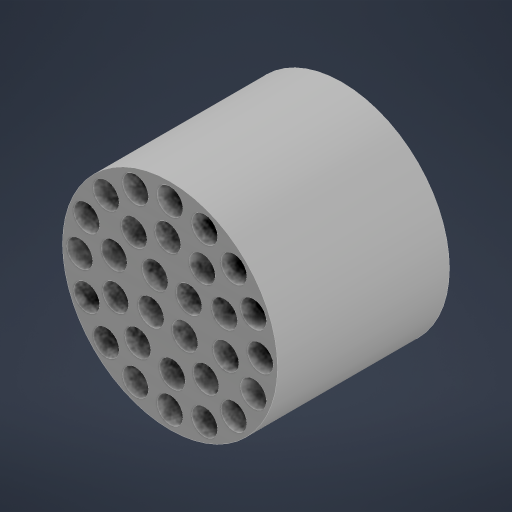
# Autodesk Inventor part: Membaranacentral
Saved by Autodesk Inventor 2024 (Build 280153000, 153)
## iProperties
Created: 2020-11-27
Part Number: Membaranacentral
Material: Plástico PET
Document SubType Name: Modeling
Designer: Tania Rios
Density: 1.541 g/cm^3
Appearance: Gris claro
Mass: 167.995 g
Surface Area: 1418.19 cm^2
Volume: 109.017 cm^3
Author: Tania Rios
Autodesk Inventor part; units mm, degrees
ref_plane "YZ Plane" through (0, 0, 0) normal (1, 0, 0) x (0, 1, 0)
ref_plane "XZ Plane" through (0, 0, 0) normal (0, 1, 0) x (-1, 0, 0)
ref_plane "XY Plane" through (0, 0, 0) normal (0, 0, 1) x (1, 0, 0)
sketch "Boceto1" plane through (0, 0, 0) normal (0, 0, 1) x (1, 0, 0)
  circle A0 centre (0, 0) radius 12.5
  circle A1 centre (0, 10.5) radius 1.5
  circle A2 centre (-4.0182, 9.7007) radius 1.5
  circle A3 centre (-7.4246, 7.4246) radius 1.5
  circle A4 centre (-9.7007, 4.0182) radius 1.5
  circle A5 centre (-10.5, 0) radius 1.5
  circle A6 centre (-9.7007, -4.0182) radius 1.5
  circle A7 centre (-7.4246, -7.4246) radius 1.5
  circle A8 centre (-4.0182, -9.7007) radius 1.5
  circle A9 centre (0, -10.5) radius 1.5
  circle A10 centre (4.0182, -9.7007) radius 1.5
  circle A11 centre (7.4246, -7.4246) radius 1.5
  circle A12 centre (9.7007, -4.0182) radius 1.5
  circle A13 centre (10.5, 0) radius 1.5
  circle A14 centre (9.7007, 4.0182) radius 1.5
  circle A15 centre (7.4246, 7.4246) radius 1.5
  circle A16 centre (4.0182, 9.7007) radius 1.5
  line L0 (0, 0) -> (19.6003, 0) construction
  line L1 (0, 0) -> (15.9307, 0) construction
  circle A17 centre (3.7502, 5.6126) radius 1.5
  circle A18 centre (-0.265, 6.745) radius 1.5
  circle A19 centre (-4.179, 5.3011) radius 1.5
  circle A20 centre (-6.4968, 1.8323) radius 1.5
  circle A21 centre (-6.333, -2.3364) radius 1.5
  circle A22 centre (-3.7502, -5.6126) radius 1.5
  circle A23 centre (0.265, -6.745) radius 1.5
  circle A24 centre (4.179, -5.3011) radius 1.5
  circle A25 centre (6.4968, -1.8323) radius 1.5
  circle A26 centre (6.333, 2.3364) radius 1.5
  circle A27 centre (2.2043, 1.7377) radius 1.5
  circle A28 centre (-1.7377, 2.2043) radius 1.5
  circle A29 centre (-2.2043, -1.7377) radius 1.5
  circle A30 centre (1.7377, -2.2043) radius 1.5
  dimension "d8" = 360
  dimension "d34" = 360
  dimension "d39" = 360
  constraints: 31 centre point, 4 end point, 2 horizontal, 1 coincident, 63 other
extrude "Extrusión1" add sketch "Boceto1" along normal mid plane 20
scale "Escala1" factors (6.8248, 6.8248, 6.8248) then translate (0, 0, 0) bodies 1
